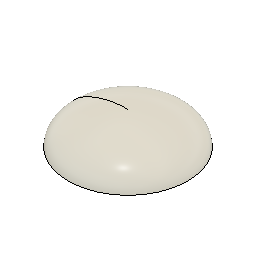
Magnetka (Autodesk Fusion 360 design; units mm, degrees)
Autodesk Fusion 360 part; units mm, degrees
sketch "Sketch1" plane through (0, 0, 0) normal (0, 0, 1) x (1, 0, 0)
  line L0 (0, 0) -> (-5.1, 0)
  line L1 (-5.1, 0) -> (-5.1, 5.1)
  line L2 (-5.1, 5.1) -> (0, 5.1)
  line L3 (0, 5.1) -> (0, 7.1)
  line L4 (0, 0) -> (0, -1)
  line L5 (0, -1) -> (-15, -1)
  spline S0 degree 5 poles (-15, -1) (-15, -0.3922) (-14.8133, 0.764) (-13.9738, 2.3202) (-11.8994, 4.069) (-8.3141, 5.7563) (-5.0579, 6.6606) (-2.5435, 7.0201) (-0.8506, 7.1) (0, 7.1) knots 0 0 0 0 0 0 0.2 0.4 0.6 0.8 1 1 1 1 1 1
  line L6 (-2.5, 7.1) -> (2.5, 7.1)
  line L7 (-15, -2.5) -> (-15, 0.5)
  line L8 (0, 2.5) -> (0, 20)
  line L9 (0, 0) -> (5.1, 0)
  spline S1 degree 5 poles (15, -1) (15, -0.3922) (14.8133, 0.764) (13.9738, 2.3202) (11.8994, 4.069) (8.3141, 5.7563) (5.0579, 6.6606) (2.5435, 7.0201) (0.8506, 7.1) (0, 7.1) knots 0 0 0 0 0 0 0.2 0.4 0.6 0.8 1 1 1 1 1 1
  line L10 (15, -2.5) -> (15, 0.5)
  line L11 (2.5, 7.1) -> (-2.5, 7.1)
  line L12 (0, -1) -> (15, -1)
  line L13 (0, 0) -> (0, -1)
  line L14 (5.1, 5.1) -> (0, 5.1)
  line L15 (0, 5.1) -> (0, 7.1)
  line L16 (5.1, 0) -> (5.1, 5.1)
  dimension "d1" = 5.1
  dimension "d2" = 5.1
  dimension "d3" = 2
  dimension "d4" = 1
  dimension "d5" = 15
  constraint coincident L0.start L4.start
  constraint horizontal L0
  constraint perpendicular L0 L1
  constraint perpendicular L1 L2
  constraint perpendicular L2 L3
  constraint perpendicular L0 L4
  constraint perpendicular L4 L5
  constraint midpoint L3.end L6
  constraint midpoint L5.end L7
  constraint symmetric L0.start L8 L4.start
  constraint symmetric L0.end L8 L9.end
  constraint symmetric L1.end L8 L14.start
  constraint symmetric L2.end L8 L3.start
  constraint symmetric L3.end L8 S0.end
  constraint symmetric L4.end L8 L5.start
  constraint symmetric L5.end L8 S1.start
  constraint symmetric L6.start L8 L6.end
  constraint symmetric L6.end L8 L6.start
  constraint symmetric L7.start L8 L10.start
  constraint symmetric L7.end L8 L10.end
  measures "d1" distance of L0.start L0.end
  measures "d2" distance of L0.end L1.end
  measures "d3" distance of L2.end L3.end
  measures "d4" distance of L0.start L4.end
  measures "d5" distance of L4.end L5.end
revolve "Revolve1" add sketch "Sketch1" angle 360 about axis through (0, 1.75, 0) along (0, 1, 0) contours L0 L1 L2 L3 L4 L5 S0 L8 L13 L15
extrude "Extrude1" cut sketch "Sketch1" along normal mid plane 10.2 contours L0 L1 L2 L9 L14 L16
named bodies: "Magnetka"
